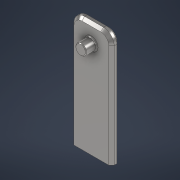
# Autodesk Inventor part: reelTab
Saved by Autodesk Inventor 2021 (Build 250183000, 183)
## iProperties
Created: 2021-06-20
Part Number: reelTab
Material: Steel, Mild
Document SubType Name: Modeling
Designer: Watchdog
Density: 7.85 g/cm^3
Appearance: Semi-Polished
Author: Watchdog
Autodesk Inventor part; units mm, degrees
ref_plane "YZ Plane" through (0, 0, 0) normal (1, 0, 0) x (0, 1, 0)
ref_plane "XZ Plane" through (0, 0, 0) normal (0, 1, 0) x (-1, 0, 0)
ref_plane "XY Plane" through (0, 0, 0) normal (0, 0, 1) x (1, 0, 0)
sketch "Sketch1" plane through (0, 0, 0) normal (0, 0, 1) x (1, 0, 0)
  line L0 (-15, 0) -> (15, 0)
  line L1 (15, 0) -> (15, 85)
  line L2 (15, 85) -> (-15, 85)
  line L3 (-15, 85) -> (-15, 0)
  point P0 (0, 0)
  dimension "d0" = 30
  dimension "d1" = 85
  dimension "d2" = 15
  dimension "d3" = 85
  constraints: 8 end point, 2 parallel, 1 horizontal, 1 perpendicular
  measures "d0" distance of L2.end L1.end
  measures "d1" distance of L1.end L0.end
  measures "d2" distance from line of point (0, 0) L3
  measures "d3" distance from line of point (0, 0) L2
extrude "Extrusion1" add sketch "Sketch1" along normal blind 6
fillet "Fillet1" radius 8 2 edges at (15, 85, 3) (-15, 85, 3)
sketch "Sketch2" plane through (0, 0, 6) normal (0, 0, 1) x (1, 0, 0)
  circle A0 centre (0, 72) radius 4
  line L0 (-15, 0) -> (15, 0) projected
  point P0 (0, 0)
  dimension "d7" = 72
  dimension "d8" = 8
  dimension "d12" = 0
  constraints: 1 centre point
  measures "d7" distance from line of L0 A0.centre
  measures "d8" diameter of A0
  measures "d12" horizontal distance of point (0, 0) A0.centre
extrude "Extrusion2" add sketch "Sketch2" along normal blind 8
fillet "Fillet2" radius 1 1 edges at (-4, 72, 6)
chamfer "Chamfer1" distance 0.5 angle 45 1 edges at (-4, 72, 14)
chamfer "Chamfer2" distance 2 angle 45 10 edges at (0, 85, 6) (-12.6569, 82.6569, 6) (-15, 38.5, 6) (12.6569, 82.6569, 6) (15, 38.5, 6) (0, 85, 0) (-12.6569, 82.6569, 0) (-15, 38.5, 0) (12.6569, 82.6569, 0) (15, 38.5, 0)
equation "\"d2\" = 0.5 * d0"
equation "\"d3\" = d1"
equation "\"d8\" = d"
equation "\"d\" = 8"
body "Solid1"
